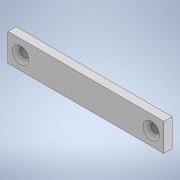
# Autodesk Inventor part: display_mount
Saved by Autodesk Inventor 2021 (Build 250183000, 183)
## iProperties
Created: 2024-09-18
Part Number: display_mount
Material: Generic
Document SubType Name: Modeling
Designer: Toby
Density: 1 g/cm^3
Appearance: Default
Author: Toby
Autodesk Inventor part; units mm, degrees
ref_plane "YZ Plane" through (0, 0, 0) normal (1, 0, 0) x (0, 1, 0)
ref_plane "XZ Plane" through (0, 0, 0) normal (0, 1, 0) x (-1, 0, 0)
ref_plane "XY Plane" through (0, 0, 0) normal (0, 0, 1) x (1, 0, 0)
sketch "Sketch1" plane through (0, 0, 0) normal (0, 0, 1) x (1, 0, 0)
  line L0 (-19.1, 3.4) -> (19.1, 3.4)
  line L1 (19.1, 3.4) -> (19.1, -3.4)
  line L2 (19.1, -3.4) -> (-19.1, -3.4)
  line L3 (-19.1, -3.4) -> (-19.1, 3.4)
  point P0 (0, 0)
  dimension "d0" = 38.2
  dimension "d1" = 6.8
  dimension "d2" = 19.1
  dimension "d3" = 3.4
  constraints: 8 end point, 2 parallel, 1 horizontal, 1 perpendicular
  measures "d0" distance of L0.start L0.end
  measures "d1" distance of L2.end L0.start
  measures "d2" distance from line of point (0, 0) L3
  measures "d3" distance from line of point (0, 0) L0
extrude "Extrusion1" add sketch "Sketch1" along normal blind 2
sketch "Sketch2" plane through (0, 0, 2) normal (0, 0, 1) x (1, 0, 0)
  line L0 (19.1, 3.4) -> (-19.1, 3.4) projected
  line L1 (-19.1, 3.4) -> (-19.1, -3.4) projected
  line L2 (19.1, -3.4) -> (19.1, 3.4) projected
  point P0 (0, 0)
  point P1 (-16, -0.1)
  point P2 (16, -0.1)
  point P3 (-16, -0.1)
  dimension "d6" = 3.5
  dimension "d7" = 3.5
  dimension "d8" = 32
  dimension "d9" = 3.1
  dimension "d10" = 3.1
  constraints: 1 coincident
  measures "d6" distance from line of point (-16, -0.1) L0
  measures "d7" distance from line of L0 point (16, -0.1)
  measures "d8" distance of point (16, -0.1) point (-16, -0.1)
  measures "d9" distance from line of L1 point (-16, -0.1)
  measures "d10" distance from line of L2 point (16, -0.1)
hole "Hole1" at (-16, -0.1, 2) at (16, -0.1, 2) direction (0, 0, -1) diameter 2 depth 4 tip angle 118 countersink diameter 4 countersink angle 90
body "Solid1"
